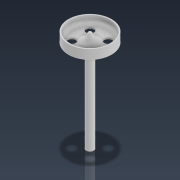
# Autodesk Inventor part: Medium turntable
Saved by Autodesk Inventor 2021.1 (Build 251245010, 245A)
## iProperties
Created: 2020-12-14
Part Number: Medium turntable
Material: 一般
Document SubType Name: Modeling
Designer: User
Density: 1 g/cm^3
Appearance: 預設
Author: User
Autodesk Inventor part; units mm, degrees
note: some values were not read from the file. Chosen so that the rebuilt part matches the saved one: direction of "孔1".
ref_plane "YZ Plane" through (0, 0, 0) normal (1, 0, 0) x (0, 1, 0)
ref_plane "XZ Plane" through (0, 0, 0) normal (0, 1, 0) x (-1, 0, 0)
ref_plane "XY Plane" through (0, 0, 0) normal (0, 0, 1) x (1, 0, 0)
sketch "草圖1" plane through (0, 0, 0) normal (0, 0, 1) x (1, 0, 0)
  line L0 (0, 0) -> (-30, 0)
  line L1 (-30, 0) -> (-30, 750)
  line L2 (-30, 750) -> (0, 750)
  line L3 (0, 750) -> (0, 0)
  line L4 (-30, 750) -> (-175, 750)
  line L5 (-175, 750) -> (-175, 825)
  line L6 (-175, 825) -> (-165, 825)
  line L7 (-165, 825) -> (-165, 760)
  line L8 (-165, 760) -> (0, 760)
  line L9 (0, 760) -> (0, 750)
  dimension "d0" = 60
  dimension "d1" = 750
  dimension "d2" = 350
  dimension "d3" = 10
  dimension "d4" = 10
  dimension "d5" = 75
  constraints: 20 end point, 6 perpendicular, 2 horizontal, 2 parallel
  measures "d0" diameter of L1 L3
  measures "d1" distance of L0.end L1.end
  measures "d2" diameter of L5 L9
  measures "d3" distance of L5.end L6.end
  measures "d4" distance between parallel lines of L8 L4
  measures "d5" distance of L4.end L5.end
revolve "迴轉1" add sketch "草圖1" angle 360 about axis through (0, 750, 0) along (0, -1, 0)
sketch "草圖2" plane through (0, 760, 0) normal (0, 1, 0) x (1, 0, 0)
  circle A0 centre (0, 0) radius 30 construction
  circle A1 centre (0, 0) radius 105 construction
  line L0 (0, 0) -> (105, 0) construction
  line L1 (74.2462, 74.2462) -> (0, 0) construction
  point P0 (-74.2462, 74.2462)
  point P1 (-74.2462, 74.2462)
  point P2 (-74.2462, -74.2462)
  point P3 (-74.2462, -74.2462)
  point P4 (74.2462, -74.2462)
  point P5 (74.2462, -74.2462)
  dimension "d7" = 210
  dimension "d8" = 45
  dimension "d11" = 360
  constraints: 5 coincident, 4 end point, 2 point on circle, 1 centre point, 1 horizontal, 9 other
  measures "d7" diameter of A1
  measures "d8" angle of L0 L1
hole "孔1" at (74.2462, 760, -74.2462) at (-74.2462, 760, -74.2462) at (-74.2462, 760, 74.2462) at (74.2462, 760, 74.2462) direction (0, -1, 0) diameter 65 depth 10
chamfer "倒角1" distance 27 angle 45 1 edges at (165, 760, 0)
sketch "草圖3" plane through (0, 0, 0) normal (0, 0, 1) x (1, 0, 0)
  line L0 (30, 0) -> (-30, 0) construction
  line L1 (-30, 0) -> (-30, 750) construction
  line L2 (-30, 750) -> (-175, 750) construction
  line L3 (-175, 750) -> (-175, 825) construction
  line L4 (-175, 825) -> (-165, 825) construction
  line L5 (-165, 825) -> (-165, 787) construction
  line L6 (-165, 787) -> (-138, 760) construction
  line L7 (-138, 760) -> (138, 760) construction
  line L8 (138, 760) -> (165, 787) construction
  line L9 (165, 787) -> (165, 825) construction
  line L10 (165, 825) -> (175, 825) construction
  line L11 (175, 825) -> (175, 750) construction
  line L12 (175, 750) -> (30, 750) construction
  line L13 (30, 750) -> (30, 0) construction
  line L14 (-138, 760) -> (138, 760) construction
  line L15 (0, 760) -> (0, 825)
  line L16 (-72.5, 760) -> (0, 760)
  line L17 (30, 750) -> (-30, 750) construction
  arc A0 (-72.5, 760) -> (-12.5, 825) centre (-91.4831, 837.7151) ccw
  line L18 (0, 825) -> (-12.5, 825)
  point P0 (0, 0)
  dimension "d23" = 72.5
  dimension "d24" = 65
  dimension "d26" = 80
  dimension "d27" = 25
  constraints: 6 end point, 2 point on circle, 1 centre point, 1 horizontal, 1 midpoint, 1 parallel, 1 point on line, 1 vertical
  measures "d23" distance of L16.start L15.start
  measures "d24" distance of L15.start L15.end
  measures "d26" radius of A0
  measures "d27" diameter of L18.end L15
revolve "迴轉2" add sketch "草圖3" angle 360 about axis through (0, 760, 0) along (0, 1, 0)
fillet "圓角1" radius 15.5 1 edges at (12.5, 825, 0)
fillet "圓角2" radius 15.5 1 edges at (165, 787, 0)
fillet "圓角3" radius 10 1 edges at (138, 760, 0)
